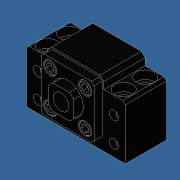
# Autodesk Inventor part: BK10 BEARING BLOCK
Saved by Autodesk Inventor 2013 SP1 (Build 170176100, 176)
## iProperties
Created: 2013-04-30
Part Number: BK10 BEARING BLOCK
Material: Aluminum 6061
Document SubType Name: Modeling
Designer: J.WASSERSTRASS
Mass: 114.295 g
Surface Area: 183.19 cm^2
Volume: 42.1753 cm^3
Density: 2.71 g/cm^3
Author: J.WASSERSTRASS
Autodesk Inventor part; units mm, degrees
ref_plane "YZ Plane" through (0, 0, 0) normal (1, 0, 0) x (0, 1, 0)
ref_plane "XZ Plane" through (0, 0, 0) normal (0, 1, 0) x (-1, 0, 0)
ref_plane "XY Plane" through (0, 0, 0) normal (0, 0, 1) x (1, 0, 0)
sketch "Sketch1" plane through (0, 0, 0) normal (0, 0, 1) x (1, 0, 0)
  line L0 (0, 0) -> (-60, 0)
  line L1 (-60, 0) -> (-60, 32.5)
  line L2 (-60, 32.5) -> (0, 32.5)
  line L3 (0, 32.5) -> (0, 0)
  line L4 (-47, 39) -> (-13, 39)
  line L5 (-13, 39) -> (-13, 32.5)
  line L6 (-13, 32.5) -> (-47, 32.5)
  line L7 (-47, 32.5) -> (-47, 39)
  point P0 (-30, 32.5)
  dimension "d0" = 60
  dimension "d1" = 39
  dimension "d2" = 34
  dimension "d3" = 32.5
  constraints: 16 end point, 4 parallel, 2 horizontal, 2 midpoint, 2 perpendicular
  measures "d0" distance of L0.start L0.end
  measures "d1" distance between parallel lines of L0 L4
  measures "d2" distance of L4.start L4.end
  measures "d3" distance of L2.end L0.start
extrude "Extrusion1" add sketch "Sketch1" along normal blind 25
sketch "Sketch2" plane through (0, 0, 25) normal (0, 0, 1) x (1, 0, 0)
  line L0 (-13, 32.5) -> (-13, 39) projected
  line L1 (-13, 39) -> (-47, 39) projected
  line L2 (-47, 39) -> (-47, 32.5) projected
  line L3 (-47, 32.5) -> (-60, 32.5) projected
  line L4 (-60, 32.5) -> (-60, 0) projected
  line L5 (-60, 0) -> (0, 0) projected
  line L6 (0, 0) -> (0, 32.5) projected
  line L7 (0, 32.5) -> (-13, 32.5) projected
  line L8 (-30, 0) -> (-30, 22) construction
  dimension "d6" = 22
  constraints: 2 end point, 1 coincident, 1 midpoint, 1 perpendicular
  measures "d6" distance from line of point (-30, 22) L5
hole "Hole1" at (-30, 22, 25) direction (0, 0, -1) diameter 20 end through all counterbore diameter 22 counterbore depth 24
sketch "Sketch3" plane through (0, 0, 25) normal (0, 0, 1) x (1, 0, 0)
  circle A0 centre (-30, 22) radius 11 construction
  line L0 (-13, 32.5) -> (-13, 39) construction
  line L1 (-13, 39) -> (-47, 39) construction
  line L2 (-47, 39) -> (-47, 32.5) construction
  line L3 (-47, 32.5) -> (-60, 32.5) construction
  line L4 (-60, 32.5) -> (-60, 0) construction
  line L5 (-60, 0) -> (0, 0) construction
  line L6 (0, 0) -> (0, 32.5) construction
  line L7 (0, 32.5) -> (-13, 32.5) construction
  line L8 (-53, 22) -> (-7, 22) construction
  line L9 (-7, 22) -> (-7, 7) construction
  line L10 (-7, 7) -> (-53, 7) construction
  line L11 (-53, 7) -> (-53, 22) construction
  dimension "d14" = 15
  dimension "d16" = 46
  constraints: 8 end point, 5 coincident, 2 parallel, 1 horizontal, 1 midpoint, 1 perpendicular
  measures "d14" distance of L8.end L9.end
  measures "d16" distance of L9.end L10.end
hole "Hole2" at (-7, 22, 25) at (-7, 7, 25) at (-53, 22, 25) at (-53, 7, 25) direction (0, 0, -1) diameter 5.5 end through all
sketch "Sketch4" plane through (-60, 32.5, 0) normal (0, 1, 0) x (1, 0, 0)
  line L0 (13, 0) -> (13, -25) construction
  line L1 (13, 0) -> (0, 0) construction
  line L2 (0, 0) -> (0, -25) construction
  line L3 (13, -25) -> (0, -25) construction
  line L4 (47, 0) -> (47, -25) construction
  line L5 (60, -25) -> (47, -25) construction
  line L6 (60, 0) -> (60, -25) construction
  line L7 (60, 0) -> (47, 0) construction
  line L8 (7, -6) -> (53, -6) construction
  line L9 (53, -6) -> (53, -19) construction
  line L10 (53, -19) -> (7, -19) construction
  line L11 (7, -19) -> (7, -6) construction
  line L12 (7, -12.5) -> (0, -12.5) construction
  line L13 (53, -12.5) -> (60, -12.5) construction
  line L14 (60, 0) -> (60, -25) construction
  dimension "d24" = 46
  dimension "d39" = 13
  constraints: 12 end point, 4 coincident, 4 midpoint, 2 parallel, 2 perpendicular, 1 collinear, 1 horizontal
  measures "d24" distance of point (7, -6) point (53, -6)
  measures "d39" distance between parallel lines of L10 L8
hole "Hole3" at (-53, 32.5, 6) at (-7, 32.5, 6) at (-53, 32.5, 19) at (-7, 32.5, 19) direction (0, -1, 0) diameter 6.6 end through all counterbore diameter 10.8 counterbore depth 5
chamfer "Chamfer1" distance 2.286 angle 45 2 edges at (-47, 39, 12.5) (-13, 39, 12.5)
chamfer "Chamfer2" distance 1.524 angle 45 2 edges at (-60, 32.5, 12.5) (0, 32.5, 12.5)
sketch "Sketch5" plane through (0, 0, 25) normal (0, 0, 1) x (1, 0, 0)
  line L0 (-1.524, 32.5) -> (0, 30.976) construction
  line L1 (-1.524, 32.5) -> (-13, 32.5) construction
  line L2 (-13, 32.5) -> (-13, 36.714) construction
  line L3 (-15.286, 39) -> (-13, 36.714) construction
  line L4 (-15.286, 39) -> (-44.714, 39) construction
  line L5 (-47, 36.714) -> (-44.714, 39) construction
  line L6 (-47, 36.714) -> (-47, 32.5) construction
  line L7 (-47, 32.5) -> (-58.476, 32.5) construction
  line L8 (-60, 30.976) -> (-58.476, 32.5) construction
  line L9 (-60, 30.976) -> (-60, 0) construction
  line L10 (-60, 0) -> (0, 0) construction
  line L11 (0, 0) -> (0, 30.976) construction
  circle A0 centre (-53, 22) radius 2.75 construction
  circle A1 centre (-7, 22) radius 2.75 construction
  circle A2 centre (-7, 7) radius 2.75 construction
  circle A3 centre (-53, 7) radius 2.75 construction
  circle A4 centre (-30, 22) radius 11 construction
  circle A5 centre (-30, 22) radius 9.5
  line L12 (-46, 6) -> (-14, 6)
  line L13 (-14, 6) -> (-14, 38)
  line L14 (-14, 38) -> (-46, 38)
  line L15 (-46, 38) -> (-46, 6)
  line L16 (-46, 6) -> (-14, 38) construction
  line L17 (-14, 6) -> (-46, 38) construction
  dimension "d40" = 32
  dimension "d42" = 19
  constraints: 12 end point, 2 midpoint, 2 parallel, 2 perpendicular, 1 centre point, 1 horizontal
  measures "d40" distance between parallel lines of L15 L13
  measures "d42" diameter of A5
extrude "Extrusion2" add sketch "Sketch5" along normal blind 5
chamfer "Chamfer3" distance 1.524 angle 45 4 edges at (-46, 38, 27.5) (-14, 38, 27.5) (-14, 6, 27.5) (-46, 6, 27.5)
sketch "Sketch7" plane through (0, 0, 30) normal (0, 0, 1) x (1, 0, 0)
  line L0 (-44.476, 6) -> (-46, 7.524) construction
  line L1 (-44.476, 6) -> (-15.524, 6) construction
  line L2 (-14, 7.524) -> (-15.524, 6) construction
  line L3 (-14, 7.524) -> (-14, 36.476) construction
  line L4 (-15.524, 38) -> (-14, 36.476) construction
  line L5 (-15.524, 38) -> (-44.476, 38) construction
  line L6 (-46, 36.476) -> (-44.476, 38) construction
  line L7 (-46, 36.476) -> (-46, 7.524) construction
  circle A0 centre (-30, 22) radius 9.5 construction
  circle A1 centre (-30, 22) radius 15 construction
  line L8 (-30, 22) -> (-45.238, 37.238) construction
  line L9 (-30, 22) -> (-14.762, 37.238) construction
  line L10 (-30, 22) -> (-14.762, 6.762) construction
  line L11 (-30, 22) -> (-45.238, 6.762) construction
  point P0 (0, 0)
  point P1 (-40.6066, 32.6066)
  point P2 (-19.3934, 32.6066)
  point P3 (-19.3934, 11.3934)
  point P4 (-40.6066, 11.3934)
  dimension "d48" = 30
  constraints: 8 end point, 4 midpoint, 4 point on circle, 4 point on line, 1 centre point, 1 perpendicular
  measures "d48" diameter of A1
hole "Hole4" at (-40.6066, 32.6066, 30) at (-19.3934, 32.6066, 30) at (-19.3934, 11.3934, 30) at (-40.6066, 11.3934, 30) direction (0, 0, -1) diameter 4.4958 depth 25.4 tip angle 118 counterbore diameter 8.001 counterbore depth 3.9878 clearance for "Socket Head Cap Screw" size "M4" standard "Ansi Metric M Profile"
sketch "Sketch8" plane through (-30, 22, 25) normal (0, 0, -1) x (-1, 0, 0)
  circle A0 centre (0, 0) radius 11 projected
  circle A1 centre (0, 0) radius 9.5 projected
  point P0 (-30, -22)
extrude "Extrusion3" add sketch "Sketch8" along normal blind 3
sketch "Sketch9" plane through (-30, 22, 22) normal (0, 0, -1) x (-1, 0, 0)
  circle A0 centre (0, 0) radius 9.5 construction
  circle A1 centre (0, 0) radius 9
  circle A2 centre (0, 0) radius 4.75
  point P0 (-30, -22)
  dimension "d59" = 18
  dimension "d61" = 9.5
  constraints: 2 centre point
  measures "d59" diameter of A1
  measures "d61" diameter of A2
extrude "Extrusion4" add sketch "Sketch9" against normal blind 12
sketch "Sketch10" plane through (-30, 22, 34) normal (0, 0, 1) x (1, 0, 0)
  circle A0 centre (0, 0) radius 4.75 projected
  circle A1 centre (0, 0) radius 9 projected
  line L0 (-4.9749, 7.5) -> (4.9749, 7.5)
  line L1 (7.5, 4.9749) -> (7.5, -4.9749)
  line L2 (4.9749, -7.5) -> (-4.9749, -7.5)
  line L3 (-7.5, -4.9749) -> (-7.5, 4.9749)
  point P0 (30, -22)
  dimension "d64" = 15
  constraints: 8 end point, 6 perpendicular, 1 horizontal, 9 other
  measures "d64" distance between parallel lines of L2 L0
extrude "Extrusion5" cut sketch "Sketch10" against normal blind 6 contours A1 L1 | L0 A1 | A1 L2 | L3 A1
sketch "Sketch11" plane through (-40.6066, 32.6066, 26.0122) normal (0, 0, 1) x (1, 0, 0)
  circle A0 centre (0, 0) radius 4.0005 construction
  circle A1 centre (0, 0) radius 2.2479 construction
  circle A2 centre (0, 0) radius 3.75
  point P0 (40.6066, -32.6066)
  dimension "d67" = 7.5
  constraints: 1 centre point
  measures "d67" diameter of A2
extrude "Extrusion6" add sketch "Sketch11" along normal blind 4
sketch "Sketch12" plane through (-40.6066, 32.6066, 30.0122) normal (0, 0, 1) x (1, 0, 0)
  circle A0 centre (0, 0) radius 3.75 projected
  line L0 (2.1374, 0.8745) -> (1.8261, -1.4138)
  line L1 (1.8261, -1.4138) -> (-0.3114, -2.2883)
  line L2 (-0.3114, -2.2883) -> (-2.1374, -0.8745)
  line L3 (-2.1374, -0.8745) -> (-1.8261, 1.4138)
  line L4 (-1.8261, 1.4138) -> (0.3114, 2.2883)
  line L5 (0.3114, 2.2883) -> (2.1374, 0.8745)
  point P0 (40.6066, -32.6066)
  dimension "d72" = 4
  constraints: 12 end point, 1 coincident, 13 other
  measures "d72" distance between parallel lines of L2 L5
extrude "Extrusion7" cut sketch "Sketch12" against normal blind 3 contours L0 L1 L2 L3 L4 L5
chamfer "Chamfer4" distance 0.508 angle 45 1 edges at (-44.3566, 32.6066, 30.0122)
pattern_circular "Circular Pattern1" count 4 over 360 about axis through (-30, 22, 22) along (0, 0, 1) of "Extrusion7", "Extrusion6", "Chamfer4"
sketch "Sketch13" plane through (0, 0, 0) normal (0, 0, -1) x (-1, 0, 0)
  circle A0 centre (30, 22) radius 10 projected
  circle A1 centre (30, 22) radius 7.1374
  circle A2 centre (30, 22) radius 5
  point P0 (0, 0)
  dimension "d81" = 14.2748
  dimension "d83" = 10
  constraints: 2 centre point, 2 coincident
  measures "d81" diameter of A1
  measures "d83" diameter of A2
extrude "Extrusion8" add sketch "Sketch13" along normal blind 1.143 contours A1
body "Solid1"
